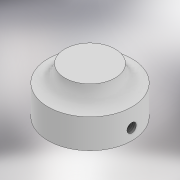
# Autodesk Inventor part: 顶垫
Saved by Autodesk Inventor 2020 (Build 240168000, 168)
## iProperties
Created: 2021-05-02
Part Number: 顶垫
Material: 常规
Document SubType Name: Modeling
Designer: Luorily
Density: 1 g/cm^3
Appearance: 默认
Author: Luorily
Autodesk Inventor part; units mm, degrees
ref_plane "XZ Plane" through (0, 0, 0) normal (0, 1, 0) x (-1, 0, 0)
ref_plane "XY Plane" through (0, 0, 0) normal (0, 0, 1) x (1, 0, 0)
sketch "草图1" plane through (0, 0, 0) normal (0, 0, 1) x (1, 0, 0)
  line L0 (-7.3546, -5.5317) -> (12.6454, -5.5317)
  line L1 (12.6454, -5.5317) -> (22.6454, -5.5317)
  line L2 (22.6454, -5.5317) -> (22.6454, 27.4683)
  line L3 (22.6454, 27.4683) -> (-7.3546, 27.4683)
  line L4 (-7.3546, 27.4683) -> (-7.3546, -5.5317)
  line L5 (12.6454, -5.5317) -> (12.6454, 8.4683)
  circle A0 centre (-7.3546, -6.5317) radius 25
  line L6 (-7.3546, -6.5317) -> (-7.3546, -5.5317)
  circle A1 centre (22.6454, 27.4683) radius 12
  point P0 (22.6454, 15.4683)
  point P1 (10.6454, 27.4683)
  point P2 (-7.3546, 18.4683)
  dimension "d6" = 50
  dimension "d0" = 20
  dimension "d1" = 10
  dimension "d2" = 33
  dimension "d3" = 30
  dimension "d4" = 14
  dimension "d7" = 24
  constraints: 14 end point, 2 perpendicular, 1 centre point, 1 coincident, 1 horizontal, 1 parallel, 1 point on line, 1 vertical, 3 other
  measures "d0" distance of L0.start L0.end
  measures "d1" distance of L0.end L1.end
  measures "d2" distance of L1.end L2.end
  measures "d3" distance of L2.end L3.end
  measures "d4" distance of L0.end L5.end
  measures "d7" diameter of A1
revolve "旋转1" add sketch "草图1" angle 360 about axis through (-7.3546, 27.4683, 0) along (0, -1, 0) contours L5 A0 L1 | L4 L3 A1 L2 L1 A0
ref_plane "工作平面1" through (22.6454, 4.9683, 0) normal (1, 0, 0) x (0, 1, 0)
sketch "草图2" plane through (22.6454, 4.9683, 0) normal (1, 0, 0) x (0, 1, 0)
  line L0 (-10.5, 20) -> (-10.5, -20) projected
  line L1 (-10.5, 0) -> (-2.5, 0)
  point P0 (-4.9683, 0)
  dimension "d9" = 8
  constraints: 2 end point, 1 coincident, 1 horizontal, 1 midpoint
  measures "d9" distance of L1.start L1.end
hole "孔1" at (22.6454, 2.4683, 0) direction (-1, 0, 0) diameter 6.647 depth 22.2 thread size "M8x1.25" designation "M8" class "6H" standard "GB Metric profile"
